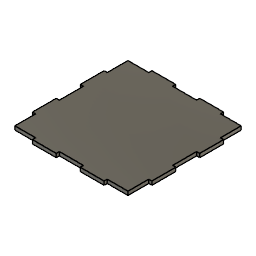
sides-1 (Autodesk Fusion 360 design; units mm, degrees)
part number: 2026-06-16-22-45-25-659
Autodesk Fusion 360 part; units mm, degrees
sketch "Sketch1" plane through (0, 0, 0) normal (0, 0, 1) x (1, 0, 0)
  line L0 (192, 6) -> (192, 186)
  line L1 (0, 186) -> (0, 6)
  line L2 (39, 192) -> (39, 186)
  line L3 (39, 186) -> (0, 186)
  line L4 (39, 192) -> (77, 192)
  line L5 (77, 192) -> (77, 186)
  line L6 (39, 186) -> (39, 192)
  line L7 (115, 192) -> (115, 186)
  line L8 (115, 186) -> (77, 186)
  line L9 (77, 186) -> (77, 192)
  line L10 (115, 192) -> (153, 192)
  line L11 (153, 192) -> (153, 186)
  line L12 (115, 186) -> (115, 192)
  line L13 (153, 192) -> (115, 192)
  line L14 (77, 192) -> (39, 192)
  line L15 (153, 186) -> (192, 186)
  line L16 (39, 0) -> (77, 0)
  line L17 (77, 0) -> (77, 6)
  line L18 (39, 6) -> (39, 0)
  line L19 (115, 0) -> (153, 0)
  line L20 (153, 0) -> (153, 6)
  line L21 (115, 6) -> (115, 0)
  line L22 (115, 0) -> (153, 0)
  line L23 (77, 6) -> (115, 6)
  line L24 (39, 6) -> (0, 6)
  line L25 (153, 6) -> (192, 6)
  line L26 (114.915, -0.085) -> (153.085, -0.085)
  line L27 (153.085, -0.085) -> (153.085, 5.915)
  line L28 (153.085, 5.915) -> (192.085, 5.915)
  line L29 (192.085, 5.915) -> (192.085, 186.085)
  line L30 (153.085, 186.085) -> (192.085, 186.085)
  line L31 (153.085, 192.085) -> (153.085, 186.085)
  line L32 (153.085, 192.085) -> (114.915, 192.085)
  line L33 (114.915, 192.085) -> (114.915, 186.085)
  line L34 (114.915, 186.085) -> (77.085, 186.085)
  line L35 (77.085, 186.085) -> (77.085, 192.085)
  line L36 (77.085, 192.085) -> (38.915, 192.085)
  line L37 (38.915, 192.085) -> (38.915, 186.085)
  line L38 (38.915, 186.085) -> (-0.085, 186.085)
  line L39 (-0.085, 186.085) -> (-0.085, 5.915)
  line L40 (38.915, 5.915) -> (-0.085, 5.915)
  line L41 (38.915, 5.915) -> (38.915, -0.085)
  line L42 (38.915, -0.085) -> (77.085, -0.085)
  line L43 (77.085, -0.085) -> (77.085, 5.915)
  line L44 (77.085, 5.915) -> (114.915, 5.915)
  line L45 (114.915, 5.915) -> (114.915, -0.085)
  dimension "d5" = 38
  dimension "d6" = 6
  dimension "d7" = 38
  dimension "d8" = 6
  dimension "d9" = 38
  dimension "d10" = 6
  dimension "d11" = 38
  dimension "d12" = 6
  dimension "d13" = 38
  dimension "d14" = 6
  dimension "d15" = 39
  dimension "d16" = 39
  dimension "d32" = 0.085
  constraint vertical L0
  constraint horizontal L13
  constraint vertical L1
  constraint vertical L2
  constraint horizontal L3
  constraint horizontal L4
  constraint vertical L5
  constraint vertical L6
  constraint vertical L7
  constraint horizontal L8
  constraint vertical L9
  constraint horizontal L10
  constraint vertical L11
  constraint vertical L12
  constraint collinear L13 L14
  constraint perpendicular L0 L15
  constraint horizontal L16
  constraint vertical L17
  constraint vertical L18
  constraint horizontal L19
  constraint vertical L20
  constraint vertical L21
  constraint perpendicular L1 L24
  constraint perpendicular L0 L25
  measures "d5" distance of L2.start L4.end
  measures "d6" distance of L2.start L2.end
  measures "d7" distance of L4.end L7.start
  measures "d8" distance of L4.end L5.end
  measures "d9" distance of L7.start L10.end
  measures "d10" distance of L7.start L7.end
  measures "d11" distance of L16.start L16.end
  measures "d12" distance of L16.start L18.start
  measures "d13" distance of L19.start L19.end
  measures "d14" distance of L19.start L21.start
  measures "d15" distance of L0 L20
  measures "d16" distance of L1 L18
extrude "Extrude1" add sketch "Sketch1" along normal blind 6 contours L0 L1 L2 L3 L4 L5 L6 L7 L8 L9 L10 L11 L12 L13 L14 L15 L16 L17 L18 L19 L20 L21 L22 L23 L24 L25
sketch "Sketch2" plane through (0, 0, 6) normal (0, 0, 1) x (-1, 0, 0)
  line L0 (-39, -6) -> (-39, 0)
  line L1 (-39, 0) -> (-77, 0)
  line L2 (-77, 0) -> (-77, -6)
  line L3 (-77, -6) -> (-115, -6)
  line L4 (-115, -6) -> (-115, 0)
  line L5 (-115, 0) -> (-153, 0)
  line L6 (-153, 0) -> (-153, -6)
  line L7 (-153, -6) -> (-192, -6)
  line L8 (-192, -6) -> (-192, -186)
  line L9 (-192, -186) -> (-153, -186)
  line L10 (-153, -186) -> (-153, -192)
  line L11 (-153, -192) -> (-115, -192)
  line L12 (-115, -192) -> (-115, -186)
  line L13 (-115, -186) -> (-77, -186)
  line L14 (-77, -186) -> (-77, -192)
  line L15 (-77, -192) -> (-39, -192)
  line L16 (-39, -192) -> (-39, -186)
  line L17 (-39, -186) -> (0, -186)
  line L18 (0, -186) -> (0, -6)
  line L19 (0, -6) -> (-39, -6)
  line L20 (-6, -186) -> (-6, -153)
  line L21 (-6, -153) -> (0, -153)
  line L22 (0, -153) -> (-6, -153)
  line L23 (-6, -115) -> (0, -115)
  line L24 (0, -115) -> (0, -153)
  line L25 (0, -115) -> (-6, -115)
  line L26 (-6, -115) -> (-6, -77)
  line L27 (-6, -77) -> (0, -77)
  line L28 (0, -77) -> (-6, -77)
  line L29 (-6, -39) -> (0, -39)
  line L30 (0, -39) -> (0, -77)
  line L31 (-6, -186) -> (-39, -186)
  line L32 (-39, -186) -> (-39, -192)
  line L33 (-6, -6) -> (-39, -6)
  line L34 (-39, -6) -> (-39, 0)
  line L35 (-6, -39) -> (-6, -6)
  line L36 (-186, -39) -> (-186, -6)
  line L37 (-186, -39) -> (-192, -39)
  line L38 (-192, -39) -> (-192, -77)
  line L39 (-186, -77) -> (-192, -77)
  line L40 (-186, -115) -> (-186, -77)
  line L41 (-192, -115) -> (-186, -115)
  line L42 (-192, -115) -> (-192, -153)
  line L43 (-186, -186) -> (-186, -153)
  line L44 (-192, -153) -> (-186, -153)
  line L45 (-186, -186) -> (-153, -186)
  line L46 (-153, -186) -> (-153, -192)
  line L47 (-153, -192) -> (-115, -192)
  line L48 (-115, -192) -> (-115, -186)
  line L49 (-115, -186) -> (-77, -186)
  line L50 (-77, -186) -> (-77, -192)
  line L51 (-77, -192) -> (-39, -192)
  line L52 (-39, -192) -> (-39, -186)
  line L53 (-39, -186) -> (0, -186)
  line L54 (0, -186) -> (0, -6)
  line L55 (0, -6) -> (-39, -6)
  line L56 (-39, -6) -> (-39, 0)
  line L57 (-39, 0) -> (-77, 0)
  line L58 (-77, 0) -> (-77, -6)
  line L59 (-77, -6) -> (-115, -6)
  line L60 (-115, -6) -> (-115, 0)
  line L61 (-115, 0) -> (-153, 0)
  line L62 (-153, 0) -> (-153, -6)
  line L63 (-153, -6) -> (-192, -6)
  line L64 (-192, -6) -> (-192, -186)
  line L65 (-192, -186) -> (-153, -186)
  line L66 (-39, 0) -> (-77, 0)
  line L67 (-77, -6) -> (-115, -6)
  line L68 (-115, 0) -> (-153, 0)
  line L69 (-153, 0) -> (-153, -6)
  line L70 (-153, -186) -> (-153, -192)
  line L71 (-153, -192) -> (-115, -192)
  line L72 (-115, -192) -> (-115, -186)
  line L73 (-39.085, -0.085) -> (-77, -0.085)
  line L74 (-39.085, -6.085) -> (-39.085, -0.085)
  line L75 (-6.085, -6.085) -> (-39.085, -6.085)
  line L76 (-6.085, -39.085) -> (-6.085, -6.085)
  line L77 (-6.085, -39.085) -> (-0.085, -39.085)
  line L78 (-0.085, -39.085) -> (-0.085, -76.915)
  line L79 (-6.085, -76.915) -> (-0.085, -76.915)
  line L80 (-6.085, -115.085) -> (-6.085, -76.915)
  line L81 (-0.085, -115.085) -> (-6.085, -115.085)
  line L82 (-0.085, -115.085) -> (-0.085, -152.915)
  line L83 (-6.085, -152.915) -> (-0.085, -152.915)
  line L84 (-6.085, -185.915) -> (-6.085, -152.915)
  line L85 (-6.085, -185.915) -> (-39.085, -185.915)
  line L86 (-39.085, -185.915) -> (-39.085, -192)
  line L87 (-186.085, -38.915) -> (-186.085, -6)
  line L88 (-186.085, -38.915) -> (-192.085, -38.915)
  line L89 (-192.085, -38.915) -> (-192.085, -77.085)
  line L90 (-186.085, -77.085) -> (-192.085, -77.085)
  line L91 (-186.085, -114.915) -> (-186.085, -77.085)
  line L92 (-192.085, -114.915) -> (-186.085, -114.915)
  line L93 (-192.085, -114.915) -> (-192.085, -153.085)
  line L94 (-192.085, -153.085) -> (-186.085, -153.085)
  line L95 (-186.085, -186.085) -> (-186.085, -153.085)
  line L96 (-186.085, -186.085) -> (-153, -186.085)
  dimension "d19" = 6
  dimension "d20" = 33
  dimension "d21" = 6
  dimension "d22" = 38
  dimension "d23" = 6
  dimension "d24" = 38
  dimension "d25" = 6
  dimension "d26" = 38
  dimension "d29" = 0
  dimension "d30" = 0.085
  dimension "d31" = 0.085
  constraint vertical L20
  constraint horizontal L21
  constraint horizontal L22
  constraint horizontal L23
  constraint vertical L24
  constraint horizontal L25
  constraint vertical L26
  constraint horizontal L27
  constraint horizontal L28
  constraint horizontal L29
  constraint vertical L30
  constraint horizontal L31
  constraint vertical L32
  constraint coincident L15.end L16.start
  constraint horizontal L33
  constraint vertical L34
  constraint coincident L0.end L1.start
  constraint perpendicular L33 L35
  constraint coincident L1.end L2.start
  constraint coincident L2.end L3.start
  constraint coincident L3.end L4.start
  constraint coincident L4.end L5.start
  constraint coincident L5.end L6.start
  constraint coincident L6.end L7.start
  constraint coincident L9.end L10.start
  constraint coincident L10.end L11.start
  constraint coincident L11.end L12.start
  measures "d19" distance of L17.end L20.start
  measures "d20" distance of L17.end L21.end
  measures "d21" distance of L21.end L20.end
  measures "d22" distance of L21.end L23.end
  measures "d23" distance of L23.end L23.start
  measures "d24" distance of L23.end L27.end
  measures "d25" distance of L27.end L26.end
  measures "d26" distance of L27.end L29.end
extrude "Extrude2" cut sketch "Sketch2" against normal blind 6 contours L0 L1 L2 L15 L16 L17 L18 L19 L20 L21 L22 L23 L24 L25 L26 L27 L28 L29 L30 L31 L32 L33 L34 L35 L51 L52 L53 L54 L55 L56 L57 L58 L66 L73 L74 L75 L76 L77 L78 L79 L80 L81 L82 L83 L84 L85 L86 | L18 L19 L29 L35 L54 L55 | L18 L23 L25 L26 L27 L28 L54 | L17 L18 L20 L21 L22 L53 L54 | L7 L8 L36 L37 L63 L64 L87 L88 | L7 L8 L63 L64 L87 L88 | L8 L39 L40 L41 L64 L90 L91 L92 | L8 L64 L90 L91 L92 | L8 L9 L43 L44 L64 L65 L94 L95 | L8 L9 L64 L65 L94 L95
extrude "Extrude3" cut 2 faces at (192, 51.6667, 2) (192, 127.6667, 4) along direction (-1, 0, 0) blind 1
extrude "Extrude4" cut 2 faces at (127.6667, 192, 4) (51.7233, 192, 2) along direction (0, -1, 0) blind 1
extrude "Extrude5" cut 2 faces at (0.085, 127.695, 2) (0.085, 51.695, 2) along direction (1, 0, 0) blind 1
extrude "Extrude6" add 1 faces at (51.7233, 0.085, 4) along direction (0, -1, 0) blind 0.085
extrude "Extrude7" cut 2 faces at (51.7233, 0, 4) (127.6667, 0, 4) along direction (0, 1, 0) blind 1
